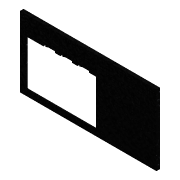
# Autodesk Inventor part: 04_OPENTRONS_Microscope_wellplate_base
Saved by Autodesk Inventor 2019.4 (Build 234330000, 330)
## iProperties
Created: 2020-11-05
Part Number: 04_OPENTRONS_Microscope_wellplate_base
Material: Generic
Document SubType Name: Modeling
Designer: diederichbenedict
Density: 1 g/cm^3
Appearance: Black
Author: diederichbenedict
Autodesk Inventor part; units mm, degrees
ref_plane "YZ Plane" through (0, 0, 0) normal (1, 0, 0) x (0, 1, 0)
ref_plane "XZ Plane" through (0, 0, 0) normal (0, 1, 0) x (-1, 0, 0)
ref_plane "XY Plane" through (0, 0, 0) normal (0, 0, 1) x (1, 0, 0)
sketch "Sketch1" plane through (0, 0, 0) normal (0, 0, 1) x (1, 0, 0)
  line L0 (-129.1, 49.6) -> (111.9, 49.6)
  line L1 (111.9, 49.6) -> (111.9, -75.4)
  line L2 (111.9, -75.4) -> (-129.1, -75.4)
  line L3 (-129.1, -75.4) -> (-129.1, 49.6)
  line L4 (-116.8, -67) -> (-68.1, -67)
  line L5 (-45.7, -67) -> (3, -67)
  line L6 (3, 18.4) -> (-45.7, 18.4)
  line L7 (-116.8, 18.5) -> (-68.1, 18.5)
  line L8 (-120.7, 14.5) -> (-120.7, -63.1)
  line L9 (-120.7, -67) -> (7.3759, -67) construction
  line L10 (7.3759, -67) -> (7.3759, 18.4) construction
  line L11 (7.3759, 18.4) -> (-120.7, 18.4) construction
  line L12 (-120.7, 18.4) -> (-120.7, -67) construction
  line L13 (4.7803, -64.4044) -> (-118.1044, -64.4044)
  line L14 (-118.1044, -64.4044) -> (-118.1044, 15.8044)
  line L15 (-118.1044, 15.8044) -> (4.7803, 15.8044)
  line L16 (4.7803, 15.8044) -> (4.7803, -64.4044)
  line L17 (-129.1, -55.4) -> (-129.1, -65.4)
  line L18 (-129.1, -75.4) -> (-119.1, -75.4) construction
  line L19 (111.9, -72.4764) -> (111.9, -32.5764) construction
  dimension "d78" = 0
  constraints: 40 end point, 7 horizontal, 6 parallel, 3 perpendicular, 3 vertical, 2 point on line, 19 other
  measures "d78" distance between parallel lines of L1 L19
extrude "Extrusion1" add sketch "Sketch1" along normal blind 2
sketch "Sketch10" plane through (0, 0, 0) normal (0, 0, -1) x (-1, 0, 0)
  line L0 (129.1, 49.6) -> (-111.9, 49.6) projected
  line L1 (-111.9, 49.6) -> (-111.9, -75.4) projected
  line L2 (-111.9, -75.4) -> (129.1, -75.4) projected
  line L3 (129.1, -75.4) -> (129.1, 49.6) projected
  line L4 (-104.9, -68.4) -> (-104.9, 42.6)
  line L5 (-104.9, 42.6) -> (122.1, 42.6)
  line L6 (122.1, 42.6) -> (122.1, -68.4)
  line L7 (122.1, -68.4) -> (-104.9, -68.4)
  line L8 (-3, 18.4) -> (45.7, 18.4)
  line L9 (-6.9, -63.1) -> (-6.9, 14.5)
  line L10 (122.1, 42.6) -> (-104.9, 42.6)
  line L11 (-104.9, 42.6) -> (-104.9, 20.8044)
  line L12 (-104.9, 20.8044) -> (122.1, 20.8044)
  line L13 (122.1, 20.8044) -> (122.1, 42.6)
  line L14 (-104.9, 20.8044) -> (-10.7803, 20.8044)
  line L15 (-10.7803, 20.8044) -> (-10.7803, -68.4)
  line L16 (-10.7803, -68.4) -> (-104.9, -68.4)
  line L17 (-104.9, -68.4) -> (-104.9, 20.8044)
  line L18 (-4.7803, 15.8044) -> (118.1044, 15.8044) projected
  line L19 (-104.9, 20.8044) -> (-12.287, 20.8044)
  line L20 (-12.287, 20.8044) -> (-12.287, -68.4)
  line L21 (-12.287, -68.4) -> (-104.9, -68.4)
  line L22 (-104.9, -68.4) -> (-104.9, 20.8044)
  line L23 (-4.7803, -64.4044) -> (-4.7803, 15.8044) projected
  point P0 (0, 0)
  dimension "d73" = 7
  dimension "d86" = 5
  dimension "d87" = 6
  constraints: 36 end point, 6 parallel, 4 horizontal, 3 perpendicular, 3 point on line, 1 vertical, 7 other
  measures "d73" distance between parallel lines of L1 L4
  measures "d86" distance between parallel lines of L18 L12
  measures "d87" distance between parallel lines of L23 L15
extrude "Extrusion7" add sketch "Sketch10" along normal blind 4 contours L3 L2 L1 L0 | L4 L12 L20 L7 | L4 L5 L6 L12 | L20 L12 L15 L7
sketch "Sketch11" plane through (0, 0, -4) normal (0, 0, -1) x (-1, 0, 0)
  circle A0 centre (124.1, -70.4) radius 1.9
  circle A1 centre (124.1, 44.6) radius 1.9
  circle A2 centre (-106.9, -15.5764) radius 3.5
  point P0 (-107.1551, -15.9364)
  constraints: 3 centre point, 6 other
hole "Hole5" at (-124.1, 44.6, -4) at (-124.1, -70.4, -4) at (106.9, -15.5764, -4) direction (0, 0, 1) diameter 4.3 depth 8 tip angle 118
fillet "Fillet2" radius 2 4 edges at (10.7803, 20.8044, -2) (10.7803, -68.4, -2) (-122.1, 20.8044, -2) (-122.1, -68.4, -2)
sketch "Sketch12" plane through (0, 0, -4) normal (0, 0, -1) x (-1, 0, 0)
  circle A0 centre (124.1, -70.4) radius 2.15 projected
  circle A1 centre (124.1, 44.6) radius 2.15 projected
  circle A2 centre (-106.9, -15.5764) radius 2.15 projected
  line L0 (129.1, -75.4) -> (129.1, 49.6) projected
  line L1 (129.1, 49.6) -> (-111.9, 49.6) projected
  line L2 (-111.9, 49.6) -> (-111.9, -75.4) projected
  line L3 (-111.9, -75.4) -> (129.1, -75.4) projected
  arc A3 (-8.7803, 20.8044) -> (-10.7803, 18.8044) centre (-8.7803, 18.8044) ccw projected
  line L4 (120.1, 20.8044) -> (-8.7803, 20.8044) projected
  arc A4 (122.1, 18.8044) -> (120.1, 20.8044) centre (120.1, 18.8044) ccw projected
  line L5 (122.1, 18.8044) -> (122.1, -66.4) projected
  arc A5 (120.1, -68.4) -> (122.1, -66.4) centre (120.1, -66.4) ccw projected
  line L6 (120.1, -68.4) -> (-8.7803, -68.4) projected
  arc A6 (-10.7803, -66.4) -> (-8.7803, -68.4) centre (-8.7803, -66.4) ccw projected
  line L7 (-10.7803, 18.8044) -> (-10.7803, -66.4) projected
  line L8 (7.5087, 20.8044) -> (25.978, 14.0821)
  line L9 (25.978, 14.0821) -> (27.478, 14.0821)
  line L10 (27.478, 14.0821) -> (27.478, 15.1324)
  line L11 (27.478, 15.1324) -> (11.8945, 20.8044)
  line L12 (120.1, 20.8044) -> (-8.7803, 20.8044) projected
  line L13 (-10.7803, 18.8044) -> (-10.7803, -66.4) projected
  line L14 (120.1, 20.8044) -> (-8.7803, 20.8044) projected
  point P0 (0, 0)
  dimension "d89" = 1.5
  dimension "d90" = 1.5
  dimension "d91" = 160
  constraints: 8 end point, 3 parallel, 2 point on line, 1 horizontal
  measures "d89" distance of L8.end L9.end
  measures "d90" distance between parallel lines of L8 L11
  measures "d91" angle of L11 L4
extrude "Extrusion9" add sketch "Sketch12" against normal blind 3 contours L4 L11 L10 L9 L8
pattern_linear "Rectangular Pattern2" count 3 spacing 30 along (-1, 0, 0) of "Extrusion9"
sketch "Sketch13" plane through (0, 0, 2) normal (0, 0, 1) x (1, 0, 0)
  line L0 (-85.978, 14.0821) -> (-67.5087, 20.8044) projected
  line L1 (-71.8945, 20.8044) -> (-87.478, 15.1324) projected
  line L2 (-55.978, 14.0821) -> (-37.5087, 20.8044) projected
  line L3 (-41.8945, 20.8044) -> (-57.478, 15.1324) projected
  line L4 (-25.978, 14.0821) -> (-7.5087, 20.8044) projected
  line L5 (-11.8945, 20.8044) -> (-27.478, 15.1324) projected
  line L6 (-116.8, 18.4) -> (3, 18.4) projected
  line L7 (-87.9063, 8.4273) -> (-67.5087, 8.4273)
  line L8 (-67.5087, 8.4273) -> (-67.5087, 18.4)
  line L9 (-67.5087, 18.4) -> (-87.9063, 18.4)
  line L10 (-87.9063, 18.4) -> (-87.9063, 8.4273)
  line L11 (-57.955, 8.4273) -> (-37.5087, 8.4273)
  line L12 (-37.5087, 8.4273) -> (-37.5087, 18.4)
  line L13 (-37.5087, 18.4) -> (-57.955, 18.4)
  line L14 (-57.955, 18.4) -> (-57.955, 8.4273)
  line L15 (-27.478, 8.4273) -> (-7.5087, 8.4273)
  line L16 (-7.5087, 8.4273) -> (-7.5087, 18.4)
  line L17 (-7.5087, 18.4) -> (-27.478, 18.4)
  line L18 (-27.478, 18.4) -> (-27.478, 8.4273)
  point P0 (0, 0)
  constraints: 24 end point, 6 parallel, 5 point on line, 3 horizontal, 3 perpendicular
extrude "Extrusion10" cut sketch "Sketch13" against normal blind 3
body "Solid1"
